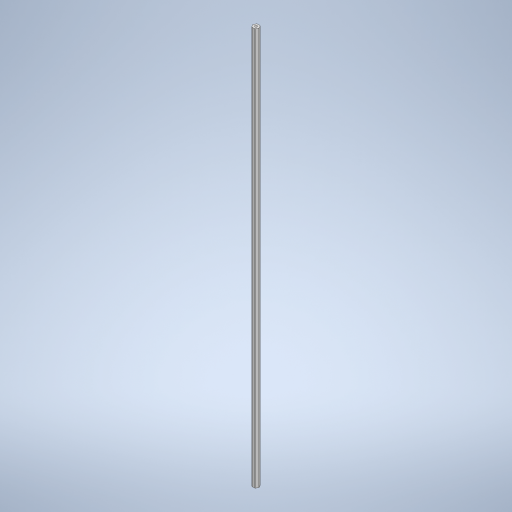
# Autodesk Inventor part: thunder hex 36in
Saved by Autodesk Inventor 2023.3 (Build 273359000, 359)
## iProperties
Created: 2023-08-25
Part Number: thunder hex 36in
Material: Generic
Document SubType Name: Modeling
Designer: jackc
Density: 1 g/cm^3
Appearance: Default
Author: jackc
Autodesk Inventor part; units mm, degrees
ref_plane "YZ Plane" through (0, 0, 0) normal (1, 0, 0) x (0, 1, 0)
ref_plane "XZ Plane" through (0, 0, 0) normal (0, 1, 0) x (-1, 0, 0)
ref_plane "XY Plane" through (0, 0, 0) normal (0, 0, 1) x (1, 0, 0)
sketch "Sketch1" plane through (0, 0, 0) normal (0, 1, 0) x (-1, 0, 0)
  line L0 (7.3323, 0) -> (3.6662, -6.35)
  line L1 (3.6662, -6.35) -> (-3.6662, -6.35)
  line L2 (-3.6662, -6.35) -> (-7.3323, 0)
  line L3 (-7.3323, 0) -> (-3.6662, 6.35)
  line L4 (-3.6662, 6.35) -> (3.6662, 6.35)
  line L5 (3.6662, 6.35) -> (7.3323, 0)
  circle A0 centre (0, 0) radius 2.5527
  circle A1 centre (0, 0) radius 6.8758
  point P0 (2.637, -6.35)
  point P1 (4.1808, -5.4587)
  point P2 (6.8178, -0.8913)
  point P3 (6.8178, 0.8913)
  point P4 (4.1808, 5.4587)
  point P5 (2.637, 6.35)
  point P6 (-2.637, 6.35)
  point P7 (-4.1808, 5.4587)
  point P8 (-6.8178, 0.8913)
  point P9 (-6.8178, -0.8913)
  point P10 (-4.1808, -5.4587)
  point P11 (-2.637, -6.35)
  dimension "d0" = 6.35
  dimension "d1" = 5.1054
  dimension "d2" = 13.7516
  constraints: 12 end point, 3 coincident, 2 centre point, 1 horizontal, 13 other
  measures "d0" distance from line of point (0, 0) L4
  measures "d1" diameter of A0
  measures "d2" diameter of A1
extrude "Extrusion1" add sketch "Sketch1" along normal blind 914.4 contours L0 A1 L1 L2 L3 L4 L5
body "Solid1"
